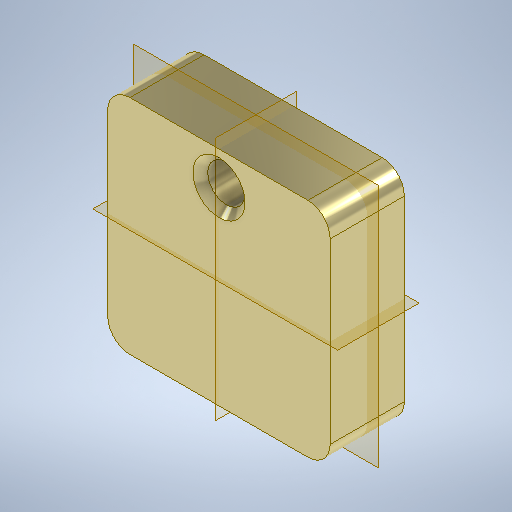
# Autodesk Inventor part: Sessao8_07_04_2025_0004_0001
Saved by Autodesk Inventor 2025.2 (Build 292293000, 293)
## iProperties
Created: 2025-04-08
Part Number: Sessao8_07_04_2025_0004_0001
Material: Ouro
Document SubType Name: Modeling
Designer: Gustavo Sousa
Density: 19.3 g/cm^3
Appearance: Ouro - Metal
Author: Gustavo Sousa
Autodesk Inventor part; units mm, degrees
sketch "Esboço1" plane through (0, 0, 0) normal (0, 0, 1) x (1, 0, 0)
  line L0 (-15, -15) -> (15, -15)
  line L1 (15, -15) -> (15, 15)
  line L2 (15, 15) -> (-15, 15)
  line L3 (-15, 15) -> (-15, -15)
  line L4 (-15, -15) -> (15, 15) construction
  line L5 (15, -15) -> (-15, 15) construction
  circle A0 centre (0, 10.49) radius 2.51
  point P0 (0, 0)
  dimension "d0" = 30
  dimension "d4" = 5.02
  dimension "d5" = 2
  constraints: 12 end point, 2 midpoint, 2 parallel, 2 perpendicular, 1 centre point, 1 horizontal, 1 vertical alignment
  measures "d0" distance of L2.end L1.end
  measures "d4" diameter of A0
  measures "d5" distance edge to line of A0 L2
extrude "Extrusão1" add sketch "Esboço1" along normal mid plane 10
fillet "Arredondamento1" radius 3 4 edges at (-15, 15, 0) (15, 15, 0) (15, -15, 0) (-15, -15, 0)
chamfer "Chanfro1" distance 1 angle 45 1 edges at (-2.51, 10.49, 5)
